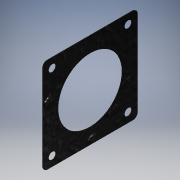
# Autodesk Inventor part: Component 22 (Cylinder Base Gasket)
Saved by Autodesk Inventor 2018 (Build 220112000, 112)
## iProperties
Created: 2023-03-25
Part Number: Component 22 (Cylinder Base Gasket)
Material: Generic
Document SubType Name: Modeling
Designer: Habib Mohamed
Density: 1 g/cm^3
Appearance: Fine Textured - Black
Author: Habib Mohamed
Autodesk Inventor part; units mm, degrees
ref_plane "YZ Plane" through (0, 0, 0) normal (1, 0, 0) x (0, 1, 0)
ref_plane "XZ Plane" through (0, 0, 0) normal (0, 1, 0) x (-1, 0, 0)
ref_plane "XY Plane" through (0, 0, 0) normal (0, 0, 1) x (1, 0, 0)
sketch "Sketch1" plane through (0, 0, 0) normal (1, 0, 0) x (0, 1, 0)
  line L0 (-18, 20) -> (18, 20)
  line L1 (20, 18) -> (20, -18)
  line L2 (18, -20) -> (-18, -20)
  line L3 (-20, -18) -> (-20, 18)
  line L4 (-20, 20) -> (20, -20) construction
  line L5 (20, 20) -> (-20, -20) construction
  circle A0 centre (16, 16) radius 1.5
  circle A1 centre (16, -16) radius 1.5
  circle A2 centre (-16, -16) radius 1.5
  circle A3 centre (-16, 16) radius 1.5
  circle A4 centre (0, 0) radius 13.5
  arc A5 (20, 18) -> (18, 20) centre (18, 18) ccw
  arc A6 (18, -20) -> (20, -18) centre (18, -18) ccw
  arc A7 (-18, 20) -> (-20, 18) centre (-18, 18) ccw
  arc A8 (-20, -18) -> (-18, -20) centre (-18, -18) ccw
  dimension "d0" = 40
  dimension "d1" = 40
  dimension "d2" = 3
  dimension "d3" = 27
  dimension "d4" = 32
  dimension "d5" = 32
  dimension "d6" = 2
  constraints: 12 end point, 12 point on line, 9 centre point, 8 point on circle, 8 tangent, 6 equal radius, 2 horizontal alignment, 2 midpoint, 2 parallel, 1 coincident, 1 horizontal, 1 perpendicular
  measures "d0" distance of L5.end L4.start
  measures "d1" distance of L4.end L5.end
  measures "d2" diameter of A0
  measures "d3" diameter of A4
  measures "d4" distance of A1.centre A0.centre
  measures "d5" distance of A3.centre A0.centre
  measures "d6" radius of A5
extrude "Extrusion1" add sketch "Sketch1" along normal blind 0.2
body "Solid1"
